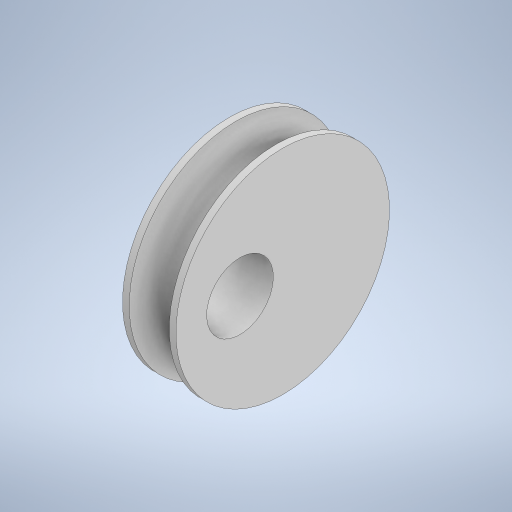
# Autodesk Inventor part: Eccentric
Saved by Autodesk Inventor 2023 (Build 270158000, 158)
## iProperties
Created: 2023-02-24
Part Number: Eccentric
Material: Generic
Document SubType Name: Modeling
Designer: tommy
Density: 1 g/cm^3
Appearance: Default
Author: tommy
Autodesk Inventor part; units mm, degrees
ref_plane "YZ Plane" through (0, 0, 0) normal (1, 0, 0) x (0, 1, 0)
ref_plane "XZ Plane" through (0, 0, 0) normal (0, 1, 0) x (-1, 0, 0)
ref_plane "XY Plane" through (0, 0, 0) normal (0, 0, 1) x (1, 0, 0)
sketch "Sketch1" plane through (0, 0, 0) normal (1, 0, 0) x (0, 1, 0)
  circle A0 centre (0, 0) radius 3.175
  circle A1 centre (0, 1.27) radius 0.9922
  line L0 (0, 0) -> (0, 1.27)
  dimension "d0" = 6.35
  dimension "d1" = 1.9844
  dimension "d2" = 1.27
  constraints: 2 centre point, 2 end point, 1 coincident, 1 vertical
  measures "d0" diameter of A0
  measures "d1" diameter of A1
  measures "d2" distance of point (0, 0) L0.end
extrude "Extrusion1" add sketch "Sketch1" along normal blind 1.5875
sketch "Sketch2" plane through (0, 0, 0) normal (0, 0, 1) x (1, 0, 0)
  line L0 (0, 3.175) -> (1.5875, 3.175) projected
  circle A0 centre (0.7937, 3.175) radius 0.5953
  line L1 (-0.3175, 0) -> (1.905, 0) projected
  point P0 (0, 0)
  dimension "d5" = 1.1906
  constraints: 1 centre point, 1 midpoint
  measures "d5" diameter of A0
revolve "Revolution1" cut sketch "Sketch2" angle 360 about axis through (-10, 0, 0) along (1, 0, 0)
body "Solid1"
